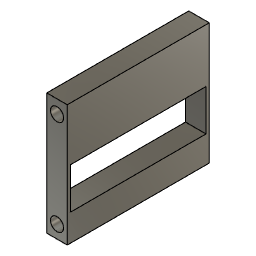
biolistener_case_v6 (Autodesk Fusion 360 design; units mm, degrees)
Autodesk Fusion 360 part; units mm, degrees
sketch "Sketch1" plane through (0, 0, 0) normal (0, 0, 1) x (1, 0, 0)
  line L0 (27.1, 17.5) -> (-25.5, 17.5)
  line L1 (-25.5, 17.5) -> (-25.5, -17.5)
  line L2 (-25.5, -17.5) -> (27.1, -17.5)
  line L3 (25.5, -19.1) -> (25.5, 19.1)
  line L4 (25.5, 17.5) -> (-25.5, -17.5) construction
  line L5 (-25.5, 17.5) -> (25.5, -17.5) construction
  line L6 (27.1, 19.1) -> (-27.1, 19.1)
  line L7 (-27.1, 19.1) -> (-27.1, -19.1)
  line L8 (-27.1, -19.1) -> (27.1, -19.1)
  line L9 (27.1, -19.1) -> (27.1, 19.1)
  line L10 (-17.5, 19.1) -> (-17.5, -19.1)
  line L11 (-19.1, 19.1) -> (-19.1, -19.1)
  line L12 (-11.5, 19.1) -> (-11.5, -19.1)
  dimension "d1" = 51
  dimension "d2" = 35
  dimension "d6" = 8
  dimension "d7" = 1.6
  dimension "d33" = -6
  constraint horizontal L0
  constraint perpendicular L0 L1
  constraint parallel L0 L2
  constraint parallel L1 L3
  constraint coincident L4 origin
  constraint coincident L5 origin
  constraint coincident L6 L10.start
  constraint coincident L8 L10.end
  constraint perpendicular L8 L10
  constraint perpendicular L6 L10
  constraint coincident L6 L3.end
  constraint coincident L4.start L3
  constraint coincident L8 L3.start
  constraint coincident L5.end L3
  constraint coincident L9 L2.end
  constraint coincident L5.end L2
  constraint coincident L9 L0.start
  constraint coincident L4.start L0
  measures "d1" distance of L1.end L5.end
  measures "d2" distance of L0.end L1.end
  measures "d6" distance of L1 L10
extrude "Extrude1" add sketch "Sketch1" against normal blind 1.6 contours L0 L2 L3 L9 | L0 L3 L6 L9 | L0 L2 L3 L12 | L0 L3 L6 L12 | L2 L3 L8 L9 | L0 L2 L10 L12 | L0 L6 L10 L12 | L2 L3 L8 L12 | L0 L2 L10 L11 | L0 L6 L10 L11 | L2 L8 L10 L12 | L2 L8 L10 L11 makes body 1
extrude "Extrude2" add sketch "Sketch1" along normal blind 10 contours L0 L3 L6 L9 | L0 L3 L6 L12 | L2 L3 L8 L9 | L0 L6 L10 L12 | L2 L3 L8 L12 | L0 L2 L10 L11 | L0 L6 L10 L11 | L2 L8 L10 L12 | L2 L8 L10 L11 bodies 1
ref_plane "WorkPlane1" through (4, 0, 10) normal (0, 0, 1) x (1, 0, 0)
sketch "Sketch2" plane through (0, 0, 10) normal (0, 0, 1) x (1, 0, 0)
  line L0 (-27.1, 19.1) -> (-27.1, -19.1)
  line L1 (-25.5, 17.5) -> (-25.5, -17.5)
  line L2 (-27.1, -19.1) -> (27.1, -19.1)
  line L3 (-25.5, -17.5) -> (27.1, -17.5)
  line L4 (27.1, 17.5) -> (-25.5, 17.5)
  line L5 (27.1, 19.1) -> (-27.1, 19.1)
  line L6 (-19.1, 19.1) -> (-19.1, -19.1)
  line L7 (-17.5, 19.1) -> (-17.5, -19.1)
  line L8 (25.5, -19.1) -> (25.5, 19.1)
  line L9 (27.1, -19.1) -> (27.1, 19.1)
extrude "Extrude3" add sketch "Sketch2" along normal blind 1.6 contours L1 L3 L4 L6 | L3 L4 L6 L7 bodies 1
extrude "Extrude4" add sketch "Sketch2" along normal blind 20 contours L0 L1 L2 L3 L4 L5 L6 | L4 L5 L6 L7 | L2 L3 L6 L7 | L4 L5 L7 L8 | L2 L3 L7 L8 | L4 L5 L8 L9 | L2 L3 L8 L9 bodies 1
ref_plane "WorkPlane2" through (0, 0, 30) normal (0, 0, 1) x (1, 0, 0)
sketch "Sketch3" plane through (0, 0, 30) normal (0, 0, 1) x (1, 0, 0)
  line L0 (-27.1, -19.1) -> (27.1, -19.1)
  line L1 (-27.1, 19.1) -> (-27.1, -19.1)
  line L2 (27.1, 19.1) -> (-27.1, 19.1)
  line L3 (27.1, 19.1) -> (27.1, -19.1)
extrude "Extrude5" add sketch "Sketch3" along normal blind 1.6 bodies 1
sketch "Sketch4" plane through (-19.1, 0, 0) normal (-1, 0, 0) x (0, -1, 0)
  line L0 (-19.1, 10) -> (-19.1, -1.6)
  line L1 (-19.1, -1.6) -> (19.1, -1.6)
  line L2 (19.1, -1.6) -> (19.1, 10)
  line L3 (19.1, 10) -> (-19.1, 10)
  line L4 (4, 0) -> (-4, 0)
  line L5 (-5, 1) -> (-5, 2)
  line L6 (-4, 3) -> (4, 3)
  line L7 (5, 2) -> (5, 1)
  arc A0 (5, 2) -> (4, 3) centre (4, 2) ccw
  arc A1 (4, 0) -> (5, 1) centre (4, 1) ccw
  arc A2 (-5, 1) -> (-4, 0) centre (-4, 1) ccw
  arc A3 (-4, 3) -> (-5, 2) centre (-4, 2) ccw
  point P0 (5, 0)
  point P1 (-5, 0)
  point P2 (5, 3)
  dimension "d20" = 10
  dimension "d21" = 3
  dimension "d22" = 1
  constraint horizontal L4
  constraint vertical L5
  constraint horizontal L6
  constraint vertical L7
  constraint coincident P2 L6
  constraint coincident P2 L7
  constraint tangent L6 A0
  constraint tangent L7 A0
  constraint coincident L4 origin
  constraint coincident P0 L4
  constraint coincident P0 L7
  constraint tangent L4 A1
  constraint tangent L7 A1
  constraint equal A0 A1
  constraint coincident P1 L4
  constraint coincident P1 L5
  constraint tangent L4 A2
  constraint tangent L5 A2
  constraint equal A0 A2
  constraint tangent L5 A3
  constraint tangent L6 A3
  constraint equal A0 A3
  measures "d20" distance of P0 P1
  measures "d21" distance of P0 P2
  measures "d22" radius of A0
extrude "Extrude6" cut sketch "Sketch4" against normal blind 1.6 contours L4 L5 L6 L7 A0 A1 A2 A3 bodies 1
chamfer "Chamfer1" distance 4 angle 45 1 edges at (-19.1, 0, 10) on bodies 1
ref_plane "WorkPlane3" through (27.1, 0, 15) normal (1, 0, 0) x (0, -1, 0)
sketch "Sketch5" plane through (27.1, 0, 0) normal (1, 0, 0) x (0, 1, 0)
  line L0 (-17.5, 30) -> (17.5, 30)
  line L1 (17.5, 30) -> (17.5, 0)
  line L2 (17.5, 0) -> (-17.5, 0)
  line L3 (-17.5, 0) -> (-17.5, 30)
  line L4 (17.5, 30) -> (-17.5, 30)
  line L5 (17.5, 0) -> (17.5, 30)
  line L6 (17.3, 0.2) -> (-17.3, 0.2)
  line L7 (-17.3, 0.2) -> (-17.3, 29.8)
  line L8 (-17.3, 29.8) -> (17.3, 29.8)
  line L9 (17.3, 29.8) -> (17.3, 0.2)
  line L10 (-17.3, 6.75) -> (17.3, 6.75)
  line L11 (-16.5, 16.75) -> (16.5, 16.75)
  line L12 (16.5, 16.75) -> (16.5, 6.75)
  line L13 (16.5, 6.75) -> (-16.5, 6.75)
  line L14 (-16.5, 6.75) -> (-16.5, 16.75)
  dimension "d27" = 0.2
  dimension "d28" = 6.75
  dimension "d29" = 33
  dimension "d30" = 10
  constraint horizontal L0
  constraint vertical L1
  constraint horizontal L2
  constraint vertical L3
  constraint equal L0 L4
  constraint equal L1 L5
  constraint coincident L7 L10.start
  constraint coincident L9 L10.end
  constraint perpendicular L9 L10
  constraint horizontal L11
  constraint vertical L12
  constraint horizontal L13
  constraint vertical L14
  constraint midpoint L10 L13
  measures "d28" distance of L2 L10
  measures "d29" distance of L11.start L11.end
  measures "d30" distance of L11.start L13.end
extrude "Extrude7" add sketch "Sketch5" against normal blind 5 separate body contours L6 L7 L9 L10 L13 | L7 L8 L9 L10 L11 L12 L14 makes body 2
extrude "Extrude8" cut sketch "Sketch1" along normal blind 16 contours L2 L8 L10 L12 bodies 1
sketch "Sketch6" plane through (-17.5, 0, 0) normal (1, 0, 0) x (0, 1, 0)
  arc A0 (4, 0) -> (5, 1) centre (4, 1) ccw
  line L0 (4, 0) -> (17.5, 0)
  line L1 (17.5, 0) -> (17.5, 11.6)
  line L2 (17.5, 11.6) -> (-17.5, 11.6)
  line L3 (-17.5, 11.6) -> (-17.5, 16)
  line L4 (-17.5, 16) -> (-19.1, 16)
  line L5 (-19.1, 16) -> (-19.1, 0)
  line L6 (-19.1, 0) -> (-4, 0)
  arc A1 (-5, 1) -> (-4, 0) centre (-4, 1) ccw
  line L7 (-5, 1) -> (-5, 2)
  arc A2 (-4, 3) -> (-5, 2) centre (-4, 2) ccw
  line L8 (-4, 3) -> (4, 3)
  arc A3 (5, 2) -> (4, 3) centre (4, 2) ccw
  line L9 (5, 2) -> (5, 1)
  line L10 (-16.1, 5) -> (-14.5, 5)
  line L11 (-14.5, 5) -> (-14.5, 10)
  line L12 (-14.5, 10) -> (-16.1, 10)
  line L13 (-16.1, 10) -> (-16.1, 5)
  line L14 (-16.1, 3) -> (-7.873, 3) construction
  line L15 (-16.1, 8.6) -> (-16.1, 3) construction
  line L16 (14.5, 8.6) -> (-16.1, 8.6) construction
  line L17 (14.5, 3) -> (14.5, 8.6) construction
  line L18 (7.873, 3) -> (14.5, 3) construction
  arc A4 (7.873, 3) -> (4, 6) centre (4, 2) ccw construction
  line L19 (-4, 6) -> (4, 6) construction
  arc A5 (-4, 6) -> (-7.873, 3) centre (-4, 2) ccw construction
  line L20 (-19.1, 0) -> (19.1, 0)
  dimension "d36" = 1.6
  dimension "d37" = 5
  dimension "d38" = -3
  dimension "d39" = 5
  constraint horizontal L10
  constraint vertical L11
  constraint horizontal L12
  constraint vertical L13
  constraint collinear L13 L15
  measures "d36" distance of L10.start L10.end
  measures "d37" distance of L10.start L12.end
  measures "d39" distance of L10 L20
extrude "Extrude9" add sketch "Sketch6" along normal blind 7 contours L10 L11 L12 L13 bodies 1
chamfer "Chamfer2" distance 6 angle 45 1 edges at (-17.5, -14.5, 7.5) on bodies 1
sketch "Sketch7" plane through (0, -17.3, 0) normal (0, -1, 0) x (1, 0, 0)
  line L0 (27.1, 0.2) -> (27.1, 29.8)
  line L1 (27.1, 29.8) -> (22.1, 29.8)
  line L2 (22.1, 29.8) -> (22.1, 0.2)
  line L3 (22.1, 0.2) -> (27.1, 0.2)
  circle A0 centre (24.6, 3.3622) radius 1.6
  line L4 (24.6, 0.2) -> (24.6, 29.8)
  circle A1 centre (24.6, 26.5676) radius 1.6
  circle A2 centre (24.6, 26.5676) radius 1.25
  circle A3 centre (24.6, 3.3622) radius 1.25
  dimension "d43" = 3.2
  dimension "d44" = 3.2
  dimension "d49" = 2.5
  dimension "d50" = 2.5
  constraint midpoint L3 L4.start
  constraint midpoint L1 L4.end
  constraint coincident A0.centre L4
  constraint coincident L4 A1.centre
  constraint concentric A1 A2
  constraint concentric A0 A3
  measures "d43" diameter of A0
  measures "d44" diameter of A1
  measures "d49" diameter of A2
  measures "d50" diameter of A3
extrude "Extrude10" cut sketch "Sketch7" against normal blind 3 contours A0 L4 A3 | A0 L4 A3 | L4 A1 A2 | L4 A1 A2 | L4 A3 | L4 A3 | L4 A2 | L4 A2 bodies 2
mirror "Mirror1" about plane through (0, 0, 0) normal (0, 1, 0) of "Extrude10"
extrude "Extrude11" cut sketch "Sketch7" along normal blind 2 contours L4 A3 | L4 A3 | L4 A2 | L4 A2 bodies 1
chamfer "Chamfer3" distance 0.9 angle 45 2 edges at (23.4346, -19.1, 27.0196) (23.4346, -19.1, 3.8142) on bodies 1
mirror "Mirror2" about plane through (0, 0, 0) normal (0, 1, 0) of 4 faces at (25.8484, -17.7333, 3.4245) (23.7729, -17.9667, 25.6303) (24.4617, -18.8, 1.5173) (23.0715, -18.8, 27.6097) on bodies 1
fillet "Fillet1" radius 1 19 edges at (-19.1, 0, -1.6) (-19.1, -19.1, 2.2) (-21.1, -19.1, 8) (-25.1, -19.1, 10) (-27.1, 0, 10) (-27.1, -19.1, 20.8) (4, -19.1, -1.6) (4, 19.1, -1.6) (-19.1, 19.1, 2.2) (-21.1, 19.1, 8) (-25.1, 19.1, 10) (-27.1, 19.1, 20.8) (0, 19.1, 31.6) (27.1, 19.1, 15) (27.1, 0, -1.6) (27.1, -19.1, 15) (0, -19.1, 31.6) (-27.1, 0, 31.6) (27.1, 0, 31.6) on bodies 1
fillet "Fillet2" radius 1.5 3 edges at (-17.5, -19.1, 8) (-14.5, -19.1, 16) (-11.5, -19.1, 8) on bodies 1
fillet "Fillet3" radius 0.5 2 edges at (-14.05, -19.1, 0) (-18.3059, -19.0786, 0) on bodies 1
hidden bodies 1
named bodies: "biolistener_case_main_body", "biolistener_case_cover"
